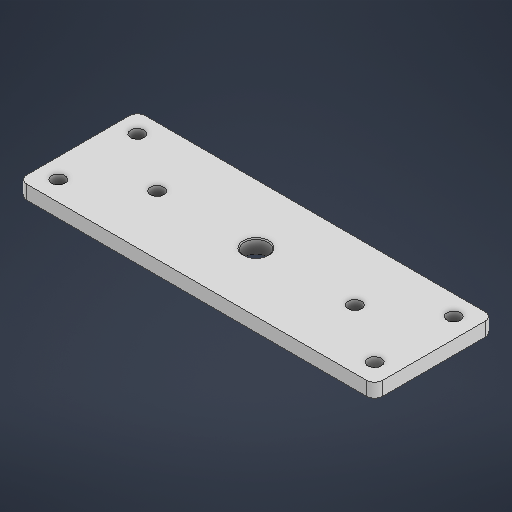
# Autodesk Inventor part: motor mount plate  for print
Saved by Autodesk Inventor 2025.2 (Build 292293000, 293)
## iProperties
Created: 2025-05-10
Part Number: motor mount plate  for print
Material: Generic
Document SubType Name: Modeling
Designer: klawy
Density: 1 g/cm^3
Appearance: Default
Author: klawy
Autodesk Inventor part; units mm, degrees
ref_plane "YZ Plane" through (0, 0, 0) normal (1, 0, 0) x (0, 1, 0)
ref_plane "XZ Plane" through (0, 0, 0) normal (0, 1, 0) x (-1, 0, 0)
ref_plane "XY Plane" through (0, 0, 0) normal (0, 0, 1) x (1, 0, 0)
sketch "Sketch1" plane through (0, 0, 0) normal (0, 1, 0) x (-1, 0, 0)
  circle A0 centre (0, 0) radius 8 construction
  circle A1 centre (0, 0) radius 3
  line L0 (45, 15) -> (-45, 15)
  line L1 (-45, 15) -> (-45, -15)
  line L2 (-45, -15) -> (45, -15)
  line L3 (45, -15) -> (45, 15)
  line L4 (0, -21) -> (0, 21) projected
  point P0 (0, 15)
  dimension "d0" = 16
  dimension "d3" = 6
  dimension "d4" = 90
  dimension "d5" = 30
  dimension "d6" = 15
  constraints: 8 end point, 2 centre point, 2 coincident, 2 parallel, 1 horizontal, 1 midpoint, 1 perpendicular, 1 point on line
  measures "d0" diameter of A0
  measures "d3" diameter of A1
  measures "d4" distance of L0.start L0.end
  measures "d5" distance of L0.end L1.end
  measures "d6" distance from line of L0 point (0, 0)
extrude "Extrusion1" add sketch "Sketch1" along normal blind 2.5 contours A1 L4 L0 L3 L2 | A1 L4 L2 L1 L0
sketch "Sketch2" plane through (0, 2.5, 0) normal (0, 1, 0) x (1, 0, 0)
  line L0 (-45, 15) -> (-45, -15) projected
  line L1 (-45, -15) -> (45, -15) projected
  line L2 (45, -15) -> (45, 15) projected
  line L3 (45, 15) -> (-45, 15) projected
  circle A0 centre (0, 0) radius 3 projected
extrude "Extrusion2" add sketch "Sketch2" along normal blind 1
sketch "Sketch7" plane through (0, 0, 0) normal (0, -1, 0) x (1, 0, 0)
  circle A0 centre (-40, 10) radius 4
  line L0 (-45, 15) -> (45, 15) projected
  line L1 (-45, -15) -> (-45, 15) projected
  circle A1 centre (40, 10) radius 4
  circle A2 centre (-40, -10) radius 4
  circle A3 centre (40, -10) radius 4
  point P0 (0, 0)
  dimension "d34" = 8
  dimension "d35" = 5
  dimension "d36" = 5
  dimension "d39" = 80
  dimension "d42" = 20
  constraints: 4 centre point, 1 horizontal, 1 vertical, 6 other
  measures "d34" diameter of A0
  measures "d35" distance from line of L0 A0.centre
  measures "d36" distance from line of L1 A0.centre
  measures "d39" distance of A0.centre A1.centre
  measures "d42" distance of A0.centre A2.centre
extrude "Extrusion4" cut sketch "Sketch7" against normal blind 1
sketch "Sketch9" plane through (0, 3.5, 0) normal (0, 1, 0) x (1, 0, 0)
  circle A0 centre (-40, -10) radius 4 construction
  point P0 (0, 0)
  constraints: 1 coincident
hole "Hole2" at (-40, 3.5, 10) direction (0, -1, 0) diameter 3.4 end through all clearance for "Socket Head Cap Screw ISO 4762" size "M3" standard "ISO"
pattern_linear "Rectangular Pattern1" count 2 spacing 20 along (0, 0, -1) count 2 spacing 80 along (1, 0, 0) of "Hole2"
chamfer "Chamfer2" distance 0.25 angle 45 1 edges at (-3, 3.5, 0)
sketch "Sketch11" plane through (0, 3.5, 0) normal (0, 1, 0) x (1, 0, 0)
  line L0 (-25, 0) -> (25, 0) construction
  point P0 (0, 0)
  point P1 (0, 0)
  dimension "d73" = 50
  constraints: 3 coincident, 2 end point, 1 horizontal, 1 midpoint
  measures "d73" distance of L0.start L0.end
hole "Hole3" at (-25, 3.5, 0) at (25, 3.5, 0) direction (0, -1, 0) diameter 3.4 end through all clearance for "Socket Head Cap Screw ISO 4762" size "M3" standard "ISO"
fillet "Fillet1" radius 2 4 edges at (-45, 1.75, 15) (45, 1.75, 15) (45, 1.75, -15) (-45, 1.75, -15)
body "Solid1"
